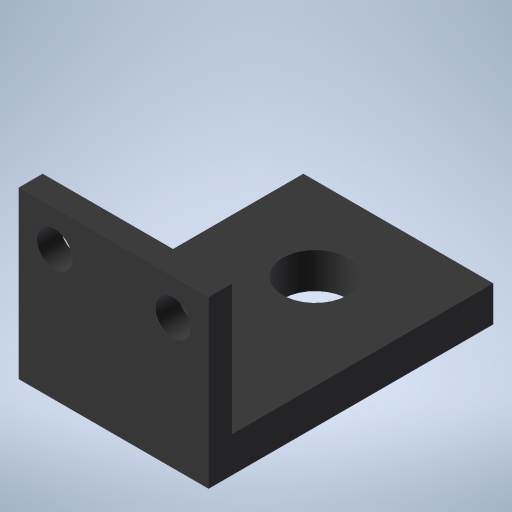
# Autodesk Inventor part: держатель вала
Saved by Autodesk Inventor 2024.2 (Build 282272000, 272)
## iProperties
Created: 2025-11-27
Part Number: держатель вала
Material: Типовые
Document SubType Name: Modeling
Designer: Zakhar
Density: 1 g/cm^3
Appearance: По умолчанию
Author: Zakhar
Autodesk Inventor part; units mm, degrees
ref_plane "YZ Plane" through (0, 0, 0) normal (1, 0, 0) x (0, 1, 0)
ref_plane "XZ Plane" through (0, 0, 0) normal (0, 1, 0) x (-1, 0, 0)
ref_plane "XY Plane" through (0, 0, 0) normal (0, 0, 1) x (1, 0, 0)
sketch "Эскиз6" plane through (0, 0, 0) normal (0, 0, 1) x (1, 0, 0)
  line L0 (0, 0) -> (-16, 0)
  line L1 (-16, 0) -> (-16, -14)
  line L2 (-16, -14) -> (0, -14)
  line L3 (0, -14) -> (0, 0)
  circle A0 centre (-3, -3) radius 1.5
  circle A1 centre (-13, -3) radius 1.5
  line L4 (0, -11) -> (-16, -11)
  line L5 (-16, -11) -> (-16, -14)
  line L6 (-16, -14) -> (0, -14)
  line L7 (0, -14) -> (0, -11)
  dimension "d42" = 16
  dimension "d43" = 14
  dimension "d44" = 3
  dimension "d45" = 3
  dimension "d46" = 3
  dimension "d47" = 3
  dimension "d48" = 3
  dimension "d49" = 3
  dimension "d50" = 3
  constraints: 16 end point, 4 parallel, 2 centre point, 2 horizontal, 2 perpendicular, 1 coincident, 1 point on line
  measures "d42" distance of L1.end L2.end
  measures "d43" distance of L0.end L1.end
  measures "d44" diameter of A1
  measures "d45" diameter of A0
  measures "d46" distance from line of L0 A1.centre
  measures "d47" distance from line of L1 A1.centre
  measures "d48" distance from line of L0 A0.centre
  measures "d49" distance from line of L3 A0.centre
  measures "d50" distance between parallel lines of L2 L4
extrude "Выдавливание8" add sketch "Эскиз6" against normal blind 2 contours L3 L4 L1 L0
extrude "Выдавливание9" add sketch "Эскиз6" against normal blind 24 contours L3 L2 L1 L4
sketch "Эскиз7" plane through (-16, -14, 0) normal (0, -1, 0) x (1, 0, 0)
  line L0 (0, 0) -> (16, 0) projected
  line L1 (16, -2) -> (0, -2) projected
  circle A0 centre (8, -17) radius 2.75
  point P0 (8, 0)
  dimension "d55" = 17
  dimension "d56" = 5.5
  constraints: 1 centre point, 1 midpoint
  measures "d55" distance of A0.centre point (8, 0)
  measures "d56" diameter of A0
extrude "Выдавливание10" cut sketch "Эскиз7" against normal blind 24
